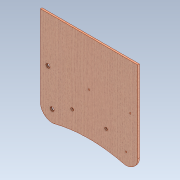
# Autodesk Inventor part: FTC Outside Panels
Saved by Autodesk Inventor 2020 (Build 240168000, 168)
## iProperties
Created: 2022-09-23
Part Number: FTC Outside Panels
Material: Wood (Oak)
Document SubType Name: Modeling
Designer: Jason
Density: 0.76 g/cm^3
Appearance: White Oak - Natural Medium Gloss
Author: Jason
Autodesk Inventor part; units mm, degrees
ref_plane "YZ Plane" through (0, 0, 0) normal (1, 0, 0) x (0, 1, 0)
ref_plane "XZ Plane" through (0, 0, 0) normal (0, 1, 0) x (-1, 0, 0)
ref_plane "XY Plane" through (0, 0, 0) normal (0, 0, 1) x (1, 0, 0)
sketch "Sketch1" plane through (0, 0, 0) normal (0, 0, 1) x (1, 0, 0)
  line L0 (40.3696, 0) -> (44.816, 0)
  line L1 (293.0054, 0) -> (287.9217, 0)
  arc A0 (0, 40.3696) -> (53.3921, 2.1581) centre (40.3696, 40.3696) ccw
  arc A1 (283.1915, 1.211) -> (333.375, 40.3696) centre (293.0054, 40.3696) ccw
  arc A2 (166.6875, 15.627) -> (44.816, 0) centre (166.3688, -464.9274) ccw
  arc A3 (287.9217, 0) -> (283.1915, 1.211) centre (166.3688, -464.9274) ccw
  arc A4 (53.3921, 2.1581) -> (44.816, 0) centre (166.3688, -464.9274) ccw
  arc A5 (287.9217, 0) -> (166.6875, 15.627) centre (166.3688, -464.9274) ccw
  line L2 (0, 40.3696) -> (0, 317.5)
  line L3 (333.375, 317.5) -> (333.375, 40.3696)
  line L4 (0, 317.5) -> (333.375, 317.5)
  line L5 (40.3696, 0) -> (293.0054, 0)
  point P0 (0, 0)
  point P1 (46.8129, 0.5175)
  dimension "d158" = 333.375
  dimension "d173" = 317.5
  constraints: 17 point on circle, 12 end point, 6 centre point, 1 horizontal, 1 perpendicular, 1 vertical
  measures "d158" distance between parallel lines of L3 L2
  measures "d173" distance between parallel lines of L4 L5
extrude "Extrusion1" add sketch "Sketch1" along normal blind 5.5563 contours A0 L2 L4 L3 A1 A5 A2
sketch "Sketch2" plane through (0, 0, 5.5563) normal (0, 0, 1) x (1, 0, 0)
  line L0 (43.8965, 34.0196) -> (47.5626, 40.3696)
  line L1 (43.8965, 46.7196) -> (47.5626, 40.3696)
  line L2 (36.5641, 46.7196) -> (43.8965, 46.7196)
  line L3 (36.5641, 34.0196) -> (43.8965, 34.0196)
  line L4 (36.5641, 46.7196) -> (32.898, 40.3696)
  line L5 (32.898, 40.3696) -> (36.5641, 34.0196)
  circle A0 centre (40.3696, 40.3696) radius 2.9337
  circle A1 centre (26.0449, 161.4785) radius 2.4066
  line L6 (0, 187.5234) -> (0, 40.3696)
  circle A2 centre (166.6875, 161.4785) radius 2.4066
  line L7 (333.375, 187.5234) -> (0, 187.5234)
  circle A3 centre (293.0054, 40.3696) radius 2.4066
  arc A4 (283.1915, 1.211) -> (333.375, 40.3696) centre (293.0054, 40.3696) ccw
  circle A5 centre (307.3301, 161.4785) radius 2.4066
  line L8 (333.375, 40.3696) -> (333.375, 187.5234)
  circle A6 centre (40.3696, 40.3696) radius 2.4066
  arc A7 (0, 40.3696) -> (46.8129, 0.5175) centre (40.3696, 40.3696) ccw
  line L9 (22.2394, 167.8285) -> (18.5732, 161.4785)
  line L10 (18.5732, 161.4785) -> (22.2394, 155.1285)
  line L11 (22.2394, 167.8285) -> (29.5718, 167.8285)
  line L12 (22.2394, 155.1285) -> (29.5718, 155.1285)
  line L13 (29.5718, 155.1285) -> (33.2379, 161.4785)
  line L14 (29.5718, 167.8285) -> (33.2379, 161.4785)
  circle A8 centre (26.0449, 161.4785) radius 2.9337
  point P0 (333.375, 40.3696)
  point P1 (283.1915, 1.211)
  point P2 (365.2681, 51.0131)
  point P3 (0, 0)
  point P4 (0, 0)
  dimension "d102" = 12.7
  dimension "d103" = 12.7
  dimension "d104" = 12.7
  dimension "d105" = 7.3323
  dimension "d106" = 7.3323
  dimension "d107" = 7.3323
  dimension "d108" = 7.3323
  dimension "d109" = 7.3323
  dimension "d110" = 7.3323
  dimension "d145" = 5.8674
  dimension "d160" = 333.375
  dimension "d161" = 12.7
  dimension "d162" = 12.7
  dimension "d163" = 12.7
  dimension "d164" = 7.3323
  dimension "d165" = 7.3323
  dimension "d166" = 7.3323
  dimension "d167" = 7.3323
  dimension "d168" = 7.3323
  dimension "d169" = 7.3323
  dimension "d170" = 5.8674
  constraints: 30 end point, 9 centre point, 4 horizontal, 4 point on circle, 1 coincident
  measures "d102" distance between parallel lines of L1 L5
  measures "d103" distance between parallel lines of L4 L0
  measures "d104" distance between parallel lines of L2 L3
  measures "d105" distance of L4.start L4.end
  measures "d106" distance of L4.end L5.end
  measures "d107" distance of L3.end L0.end
  measures "d108" distance of L5.end L3.end
  measures "d109" distance of L1.start L0.end
  measures "d110" distance of L4.start L2.end
  measures "d145" diameter of A0
  measures "d160" distance between parallel lines of L8 L6
  measures "d161" distance between parallel lines of L14 L10
  measures "d162" distance between parallel lines of L9 L13
  measures "d163" distance between parallel lines of L11 L12
  measures "d164" distance of L9.start L9.end
  measures "d165" distance of L9.end L10.end
  measures "d166" distance of L12.end L14.end
  measures "d167" distance of L10.end L12.end
  measures "d168" distance of L14.start L14.end
  measures "d169" distance of L9.start L11.end
  measures "d170" diameter of A8
extrude "Extrusion2" cut sketch "Sketch2" against normal through all contours L3 L5 L4 L2 L1 L0 | A0 | A1 | A2 | A3 | A5 | A6 | L11 L14 L13 L12 L10 L9 | A8
sketch "Sketch6" plane through (0, 0, 5.5563) normal (0, 0, 1) x (1, 0, 0)
  ellipse E0 centre (224.6212, 89.9867) end of major axis (224.6174, 91.9867) minor radius 2
  ellipse E1 centre (224.6212, 57.9868) end of major axis (224.6139, 59.9867) minor radius 2
  line L0 (292.9982, 40.3696) -> (224.6212, 40.3696)
  line L1 (224.6212, 40.3696) -> (224.6212, 57.9868)
  ellipse E2 centre (108.7157, 89.9867) end of major axis (108.7119, 91.9867) minor radius 2
  ellipse E3 centre (108.7466, 57.9868) end of major axis (108.7392, 59.9867) minor radius 2
  line L2 (108.7466, 40.2597) -> (108.7466, 57.8769)
  circle A0 centre (224.6521, 73.9867) radius 4.699
  circle A1 centre (108.7466, 73.9867) radius 4.699
  line L3 (40.3696, 40.2597) -> (108.7466, 40.2597)
  circle A2 centre (293.0054, 40.3696) radius 2.4066 projected
  point P0 (0, 0)
  dimension "d147" = 17.6171
  dimension "d150" = 17.6171
  dimension "d152" = 9.398
  dimension "d153" = 9.398
  dimension "d171" = 31.9999
  dimension "d172" = 31.9999
  constraints: 8 end point, 2 centre point, 2 horizontal, 1 coincident, 1 perpendicular, 1 vertical, 8 other
  measures "d147" distance of L0.end L1.end
  measures "d150" distance of L2.start L2.end
  measures "d152" diameter of A0
  measures "d153" diameter of A1
  measures "d171" distance of point (108.716, 89.987) point (108.747, 57.987)
  measures "d172" distance of L1.end point (224.621, 89.987)
extrude "Extrusion7" cut sketch "Sketch6" against normal through all contours A0 | A1
body "Solid1"
